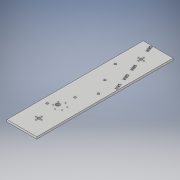
# Autodesk Inventor part: testPart_chassis2
Saved by Autodesk Inventor 2019 (Build 230136000, 136)
## iProperties
Created: 2019-09-17
Part Number: testPart_chassis2
Material: Generic
Document SubType Name: Modeling
Designer: shrey
Density: 1 g/cm^3
Appearance: Default
Author: shrey
Autodesk Inventor part; units mm, degrees
ref_plane "YZ Plane" through (0, 0, 0) normal (1, 0, 0) x (0, 1, 0)
ref_plane "XZ Plane" through (0, 0, 0) normal (0, 1, 0) x (-1, 0, 0)
ref_plane "XY Plane" through (0, 0, 0) normal (0, 0, 1) x (1, 0, 0)
sketch "Sketch1" plane through (0, 0, 0) normal (0, 1, 0) x (-1, 0, 0)
  line L0 (-44.45, -203.2) -> (44.45, -203.2)
  line L1 (44.45, -203.2) -> (44.45, 203.2)
  line L2 (44.45, 203.2) -> (-44.45, 203.2)
  line L3 (-44.45, 203.2) -> (-44.45, -203.2)
  line L4 (-44.45, -203.2) -> (44.45, 203.2) construction
  line L5 (44.45, -203.2) -> (-44.45, 203.2) construction
  line L6 (0, 203.2) -> (0, -203.2) construction
  line L7 (0, 0) -> (44.45, 0) construction
  line L8 (0, -203.2) -> (0, 203.2) construction
  line L9 (0, 152.4) -> (7.112, 152.4) construction
  line L10 (0, -152.4) -> (0, -203.2) construction
  circle A0 centre (0, -152.4) radius 4
  circle A1 centre (0, -152.4) radius 8 construction
  line L11 (0, 152.4) -> (-44.45, 152.4) construction
  line L12 (-44.45, 152.4) -> (-44.45, 88.9)
  line L13 (-44.45, 88.9) -> (0, 88.9) construction
  line L14 (0, 88.9) -> (0, 152.4) construction
  circle A2 centre (0, 88.9) radius 7.112 construction
  circle A3 centre (7.112, 88.9) radius 5.9944
  circle A4 centre (0, 88.9) radius 15.494 construction
  circle A5 centre (0, 104.394) radius 1.5
  circle A6 centre (0, 88.9) radius 15.494 construction
  circle A7 centre (-13.4182, 96.647) radius 1.5
  circle A8 centre (0, 88.9) radius 15.494 construction
  circle A9 centre (-13.4182, 81.153) radius 1.5
  circle A10 centre (0, 88.9) radius 15.494 construction
  circle A11 centre (0, 73.406) radius 1.5
  circle A12 centre (0, 88.9) radius 15.494 construction
  circle A13 centre (13.4182, 81.153) radius 1.5
  circle A14 centre (0, 88.9) radius 15.494 construction
  circle A15 centre (13.4182, 96.647) radius 1.5
  circle A16 centre (0, -144.4) radius 1.85
  circle A17 centre (-8, -152.4) radius 1.85
  circle A18 centre (0, -160.4) radius 1.85
  circle A19 centre (8, -152.4) radius 1.85
  circle A20 centre (0, 152.4) radius 4
  circle A21 centre (0, 152.4) radius 8 construction
  circle A22 centre (0, 160.4) radius 1.85
  circle A23 centre (0, 152.4) radius 8 construction
  circle A24 centre (-8, 152.4) radius 1.85
  circle A25 centre (0, 152.4) radius 8 construction
  circle A26 centre (0, 144.4) radius 1.85
  circle A27 centre (0, 152.4) radius 8 construction
  circle A28 centre (8, 152.4) radius 1.85
  line L15 (-88.9, 44.45) -> (0, 44.45) construction
  line L16 (0, 44.45) -> (0, -44.45) construction
  line L17 (0, -44.45) -> (-88.9, -44.45) construction
  line L18 (-88.9, -44.45) -> (-88.9, 44.45) construction
  line L19 (-88.9, 44.45) -> (0, -44.45) construction
  line L20 (0, 44.45) -> (-88.9, -44.45) construction
  circle A29 centre (0, 44.45) radius 2.9766
  circle A30 centre (0, -44.45) radius 2.9766
  line L21 (44.45, -203.2) -> (25.4, -203.2)
  line L22 (25.4, -203.2) -> (25.4, -101.6) construction
  line L23 (25.4, -101.6) -> (44.45, -101.6) construction
  line L24 (44.45, -101.6) -> (44.45, -203.2)
  circle A31 centre (25.9021, -101.6) radius 3.175
  circle A32 centre (25.9021, 101.6) radius 3.175
  line L25 (-44.45, -17.5714) -> (-25.4, -17.5714) construction
  line L26 (-25.4, -17.5714) -> (-25.4, 31.4423) construction
  line L27 (-25.4, 31.4423) -> (-44.45, 31.4423) construction
  line L28 (-44.45, 31.4423) -> (-44.45, -17.5714)
  circle A33 centre (-25.4, 0) radius 3.175
  line L29 (-44.45, -203.2) -> (0, -203.2)
  line L30 (-44.45, 0) -> (-44.45, -203.2)
  line L31 (-44.45, -203.2) -> (19.05, -203.2)
  line L32 (19.05, -203.2) -> (19.05, -25.4) construction
  line L33 (19.05, -25.4) -> (-44.45, -25.4) construction
  line L34 (-44.45, -25.4) -> (-44.45, -203.2)
  line L35 (19.05, -203.2) -> (-44.45, -25.4) construction
  line L36 (-44.45, -25.4) -> (-38.0428, -43.3402) construction
  line L37 (-30.3832, -55.3489) -> (-36.3634, -57.4842)
  line L38 (-36.3634, -57.4842) -> (-42.7694, -39.5436)
  line L39 (-42.7694, -39.5436) -> (-36.7892, -37.4083)
  line L40 (-36.7892, -37.4083) -> (-30.3832, -55.3489)
  line L41 (-41.2178, -33.8152) -> (-34.8678, -52.8652) construction
  line L42 (-34.8678, -33.8152) -> (-41.2178, -52.8652) construction
  line L43 (-23.549, -93.3646) -> (-29.955, -75.424)
  line L44 (-17.5688, -91.2293) -> (-23.549, -93.3646)
  line L45 (-23.9748, -73.2887) -> (-17.5688, -91.2293)
  line L46 (-29.955, -75.424) -> (-23.9748, -73.2887)
  line L47 (-10.7346, -129.245) -> (-17.1406, -111.3044)
  line L48 (-4.7544, -127.1096) -> (-10.7346, -129.245)
  line L49 (-11.1604, -109.169) -> (-4.7544, -127.1096)
  line L50 (-17.1406, -111.3044) -> (-11.1604, -109.169)
  line L51 (2.0798, -165.1253) -> (-4.3262, -147.1847)
  line L52 (8.06, -162.99) -> (2.0798, -165.1253)
  line L53 (1.654, -145.0494) -> (8.06, -162.99)
  line L54 (-4.3262, -147.1847) -> (1.654, -145.0494)
  line L55 (14.8942, -201.0057) -> (8.4882, -183.0651)
  line L56 (20.8744, -198.8704) -> (14.8942, -201.0057)
  line L57 (14.4684, -180.9298) -> (20.8744, -198.8704)
  line L58 (8.4882, -183.0651) -> (14.4684, -180.9298)
  dimension "d17" = 16
  dimension "d26" = 14.224
  dimension "d28" = 30.988
  dimension "d40" = 16
  dimension "d0" = 406.4
  dimension "d1" = 88.9
  dimension "d2" = 152.4
  dimension "d16" = 8
  dimension "d24" = 44.45
  dimension "d25" = 63.5
  dimension "d27" = 11.9888
  dimension "d29" = 3
  dimension "d32" = 360
  dimension "d34" = 3.7
  dimension "d37" = 360
  dimension "d39" = 8
  dimension "d41" = 3.7
  dimension "d44" = 360
  dimension "d63" = 88.9
  dimension "d64" = 5.9531
  dimension "d65" = 5.9531
  dimension "d71" = 101.6
  dimension "d72" = 19.05
  dimension "d73" = 6.35
  dimension "d74" = 19.05
  dimension "d75" = 6.35
  dimension "d81" = 177.8
  dimension "d82" = 63.5
  dimension "d83" = 19.05
  dimension "d84" = 6.35
  dimension "d85" = 19.05
  dimension "d88" = 38.1
  constraints: 118 end point, 22 centre point, 14 parallel, 11 coincident, 9 point on line, 8 horizontal, 7 midpoint, 7 perpendicular, 5 vertical alignment, 4 symmetric about line, 3 horizontal alignment, 1 collinear, 111 other
  measures "d0" distance of L0.end L1.end
  measures "d1" distance of L1.end L2.end
  measures "d2" distance of L7.start point (0, 152.4)
  measures "d16" diameter of A0
  measures "d24" distance of L9.start L11.end
  measures "d25" distance of L11.end L12.end
  measures "d27" diameter of A3
  measures "d29" diameter of A5
  measures "d34" diameter of A16
  measures "d39" diameter of A20
  measures "d41" diameter of A22
  measures "d63" distance of L17.end L15.start
  measures "d64" diameter of A29
  measures "d65" diameter of A30
  measures "d71" distance of L21.end L22.end
  measures "d72" distance of L22.end L23.end
  measures "d73" diameter of A31
  measures "d74" distance of L25.start L25.end
  measures "d75" diameter of A33
  measures "d81" distance of L31.end L32.end
  measures "d82" distance of L32.end L33.end
  measures "d83" distance of L33.end L36.end
  measures "d84" distance of L38.end L39.end
  measures "d85" distance of L37.end L38.end
  measures "d88" distance of L37.end L43.start
extrude "Extrusion8" add sketch "Sketch1" along normal blind 6.35 contours L3 L2 L1 L0 | A0 L51 L54 A16 L53 L52 A18
body "Solid8"
